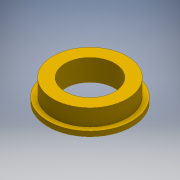
# Autodesk Inventor part: ベアリング　m4　フランジ付き
Saved by Autodesk Inventor 2016 (Build 200138000, 138)
## iProperties
Created: 2016-01-12
Part Number: ベアリング　m4　フランジ付き
Material: 一般
Document SubType Name: Modeling
Designer: Takumi
Density: 4.68151 g/cm^3
Appearance: ゴールド
Mass: 1.15 g
Surface Area: 4.13936 cm^2
Volume: 0.245647 cm^3
Author: Takumi
Autodesk Inventor part; units mm, degrees
ref_plane "YZ Plane" through (0, 0, 0) normal (1, 0, 0) x (0, 1, 0)
ref_plane "XZ Plane" through (0, 0, 0) normal (0, 1, 0) x (-1, 0, 0)
ref_plane "XY Plane" through (0, 0, 0) normal (0, 0, 1) x (1, 0, 0)
sketch "スケッチ1" plane through (0, 0, 0) normal (0, 0, 1) x (1, 0, 0)
  circle A0 centre (0, 0) radius 6
  circle A1 centre (0, 0) radius 4
  circle A2 centre (0, 0) radius 6.8
  dimension "d0" = 12
  dimension "d1" = 8
  dimension "d3" = 13.6
  constraints: 3 centre point, 3 coincident
  measures "d0" diameter of A0
  measures "d1" diameter of A1
  measures "d3" diameter of A2
extrude "押し出し1" add sketch "スケッチ1" along normal blind 3.5 contours A0
extrude "押し出し2" add sketch "スケッチ1" along normal blind 0.8 contours A2
